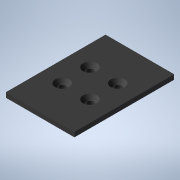
# Autodesk Inventor part: caster adapter for mobile afl
Saved by Autodesk Inventor 2020 (Build 240168000, 168)
## iProperties
Created: 2022-07-12
Part Number: caster adapter for mobile afl
Material: Generic
Document SubType Name: Modeling
Designer: Beaucage
Density: 1 g/cm^3
Appearance: Default
Author: Beaucage
Autodesk Inventor part; units mm, degrees
ref_plane "YZ Plane" through (0, 0, 0) normal (1, 0, 0) x (0, 1, 0)
ref_plane "XZ Plane" through (0, 0, 0) normal (0, 1, 0) x (-1, 0, 0)
ref_plane "XY Plane" through (0, 0, 0) normal (0, 0, 1) x (1, 0, 0)
sketch "Sketch1" plane through (0, 0, 0) normal (0, 1, 0) x (-1, 0, 0)
  line L0 (0, 0) -> (62.484, 0)
  line L1 (62.484, 0) -> (62.484, -90.932)
  line L2 (62.484, -90.932) -> (0, -90.932)
  line L3 (0, -90.932) -> (0, 0)
  dimension "d0" = 62.484
  dimension "d1" = 90.932
  constraints: 8 end point, 2 parallel, 1 horizontal, 1 perpendicular
  measures "d0" distance of L1.end L2.end
  measures "d1" distance of L0.end L1.end
extrude "Extrusion1" add sketch "Sketch1" along normal blind 4.318
sketch "Sketch3" plane through (0, 0, 0) normal (0, -1, 0) x (1, 0, 0)
  line L0 (0, 0) -> (0, -90.932) projected
  line L1 (-62.484, -90.932) -> (-62.484, 0) projected
  line L2 (-62.484, 0) -> (0, 0) projected
  line L3 (0, -90.932) -> (-62.484, -90.932) projected
  line L4 (-9.017, -23.241) -> (-53.467, -23.241)
  line L5 (-53.467, -23.241) -> (-53.467, -67.691)
  line L6 (-53.467, -67.691) -> (-9.017, -67.691)
  line L7 (-9.017, -67.691) -> (-9.017, -23.241)
  line L8 (-9.017, -23.241) -> (-53.467, -67.691) construction
  line L9 (-53.467, -23.241) -> (-9.017, -67.691) construction
  point P0 (-31.242, -45.466)
  dimension "d13" = 44.45
  dimension "d14" = 44.45
  constraints: 12 end point, 2 midpoint, 2 parallel, 1 horizontal, 1 perpendicular
  measures "d13" distance of L6.end L5.end
  measures "d14" distance of L5.end L4.end
extrude "Extrusion2" add sketch "Sketch3" along normal blind 6.35 contours L7 L6 L5 L4
sketch "Sketch2" plane through (0, 4.318, 0) normal (0, 1, 0) x (1, 0, 0)
  line L0 (-62.484, 90.932) -> (-62.484, 0) projected
  line L1 (-62.484, 45.466) -> (0, 45.466)
  line L2 (0, 90.932) -> (-62.484, 90.932) projected
  line L3 (-31.242, 90.932) -> (-31.242, 0)
  line L4 (-62.484, 0) -> (0, 0) projected
  line L5 (-18.542, 32.766) -> (-43.942, 32.766)
  line L6 (-43.942, 32.766) -> (-43.942, 58.166)
  line L7 (-43.942, 58.166) -> (-18.542, 58.166)
  line L8 (-18.542, 58.166) -> (-18.542, 32.766)
  line L9 (-18.542, 32.766) -> (-43.942, 58.166) construction
  line L10 (-43.942, 32.766) -> (-18.542, 58.166) construction
  point P0 (-31.242, 45.466)
  dimension "d4" = 25.4
  dimension "d5" = 25.4
  constraints: 16 end point, 6 midpoint, 2 horizontal, 2 parallel, 1 perpendicular
  measures "d4" distance of L6.end L7.end
  measures "d5" distance of L5.end L6.end
hole "Hole1" at (-18.542, 4.318, -32.766) at (-43.942, 4.318, -32.766) at (-18.542, 4.318, -58.166) at (-43.942, 4.318, -58.166) direction (0, -1, 0) diameter 6.7564 depth 25.4 tip angle 118 countersink diameter 12.8778 countersink angle 82 clearance for "Flat Head Machine Screw (82)" size "1/4" standard "Ansi Unified Screw Threads"
fillet "Fillet1" radius 3.175 8 edges at (-31.242, 0, -23.241) (-31.242, -6.35, -23.241) (-31.242, -6.35, -67.691) (-31.242, 0, -67.691) (-9.017, 0, -45.466) (-53.467, 0, -45.466) (-53.467, -6.35, -45.466) (-9.017, -6.35, -45.466)
body "Solid1"
